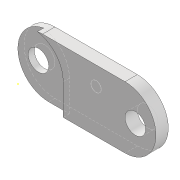
# Autodesk Inventor part: GripP3
Saved by Autodesk Inventor 2021 (Build 250183000, 183)
## iProperties
Created: 2022-09-30
Part Number: GripP3
Material: Generic
Document SubType Name: Modeling
Designer: brian
Density: 1 g/cm^3
Appearance: Default
Author: brian
Autodesk Inventor part; units mm, degrees
ref_plane "YZ Plane" through (0, 0, 0) normal (1, 0, 0) x (0, 1, 0)
ref_plane "XZ Plane" through (0, 0, 0) normal (0, 1, 0) x (-1, 0, 0)
ref_plane "XY Plane" through (0, 0, 0) normal (0, 0, 1) x (1, 0, 0)
sketch "Sketch1" plane through (0, 0, 0) normal (0, 0, 1) x (1, 0, 0)
  line L0 (15, 0) -> (55, 0)
  line L1 (70, 15) -> (70, 15)
  line L2 (55, 30) -> (15, 30)
  line L3 (0, 15) -> (0, 15)
  circle A0 centre (10, 15) radius 5
  circle A1 centre (60, 15) radius 5
  arc A2 (70, 15) -> (55, 30) centre (55, 15) ccw
  arc A3 (55, 0) -> (70, 15) centre (55, 15) ccw
  arc A4 (0, 15) -> (15, 0) centre (15, 15) ccw
  arc A5 (15, 30) -> (0, 15) centre (15, 15) ccw
  point P0 (0, 0)
  point P1 (70, 0)
  point P2 (70, 30)
  point P3 (0, 15)
  dimension "d1" = 30
  dimension "d14" = 10
  dimension "d15" = 10
  dimension "d16" = 10
  dimension "d17" = 50
  dimension "d18" = 15
  dimension "d21" = 15
  constraints: 8 end point, 8 point on circle, 8 tangent, 6 centre point, 6 point on line, 4 equal radius, 2 parallel, 1 horizontal, 1 perpendicular
  measures "d1" distance of point (70, 0) point (70, 30)
  measures "d14" diameter of A0
  measures "d15" distance from line of L3 A0.centre
  measures "d16" distance from line of A1.centre L1
  measures "d17" distance of A1.centre A0.centre
  measures "d18" radius of A2
  measures "d21" distance from line of L0 A1.centre
extrude "Extrusion1" add sketch "Sketch1" along normal blind 3
sketch "Sketch3" plane through (0, 0, 3) normal (0, 0, 1) x (1, 0, 0)
  arc A0 (55, 0) -> (55, 30) centre (55, 15) ccw projected
  line L0 (55, 30) -> (15, 30) projected
  arc A1 (15, 30) -> (15, 0) centre (15, 15) ccw projected
  line L1 (15, 0) -> (55, 0) projected
  circle A2 centre (60, 15) radius 5 projected
  circle A3 centre (10, 15) radius 5 projected
  line L2 (55, 30) -> (15, 30) projected
  line L3 (25, 30) -> (25, 0)
  circle A4 centre (10, 15) radius 15
  circle A5 centre (10, 12) radius 15
  point P0 (0, 0)
  point P1 (12.5, 29.7902)
  point P2 (25, 15)
  dimension "d24" = 15
  dimension "d27" = 3
  constraints: 2 centre point, 2 end point, 2 point on line, 2 tangent, 1 coincident, 1 perpendicular
  measures "d24" distance from line of A3.centre L3
  measures "d27" distance of A3.centre A5.centre
sketch "Sketch4" plane through (0, 0, 3) normal (0, 0, 1) x (1, 0, 0)
  point P0 (0, 0)
extrude "Extrusion3" add sketch "Sketch3" along normal blind 3 contours L1 L3 L0 A0 | L3 A4 A1 L0
sketch "Sketch5" plane through (0, 0, 0) normal (0, 0, -1) x (-1, 0, 0)
  circle A0 centre (-60, 15) radius 5 projected
  circle A1 centre (-10, 15) radius 5 projected
  circle A2 centre (-40, 15) radius 2.5
  line L0 (-25, 0) -> (-25, 15) projected
  point P0 (0, 0)
  dimension "d30" = 5
  dimension "d33" = 35
  dimension "d34" = 10
  dimension "d36" = 15
  constraints: 1 centre point, 1 horizontal alignment
  measures "d30" diameter of A2
  measures "d33" distance from line of L0 A0.centre
  measures "d34" diameter of A0
  measures "d36" distance of A2.centre L0.end
extrude "Extrusion4" cut sketch "Sketch5" against normal blind 0.1 contours A2
sketch "Sketch6" plane through (0, 0, 6) normal (0, 0, 1) x (1, 0, 0)
  circle A0 centre (40, 15) radius 2.5 projected
  point P0 (0, 0)
extrude "Extrusion5" cut sketch "Sketch6" against normal blind 0.1
equation "\"d1\" = d0"
equation "\"d14\" = d6"
equation "\"d15\" = d14"
equation "\"d16\" = d15"
equation "\"d18\" = 0.5 * d1"
equation "\"d21\" = 0.5 * d1"
equation "\"d19\" = d11"
equation "\"d24\" = 0.5 * d0"
equation "\"d27\" = 0.1 * d0"
equation "\"d25\" = d11"
equation "\"d36\" = 0.5 * d33 - 0.25 * d34"
equation "\"d6\" = 10"
equation "\"d11\" = 3"
equation "\"d0\" = 30"
body "Solid1"
